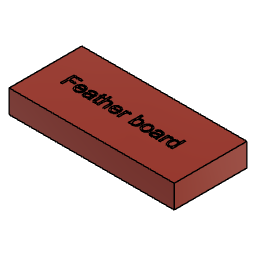
Feather board v1 (Autodesk Fusion 360 design; units mm, degrees)
Autodesk Fusion 360 part; units mm, degrees
sketch "Sketch1" plane through (0, 0, 0) normal (0, 0, 1) x (1, 0, 0)
  line L0 (0, 0) -> (50, 0)
  line L1 (50, 0) -> (50, 22)
  line L2 (50, 22) -> (0, 22)
  line L3 (0, 22) -> (0, 0)
  dimension "d1" = 50
  dimension "d2" = 22
  constraint horizontal L0
  constraint vertical L1
  constraint horizontal L2
  constraint vertical L3
  constraint coincident L0.start L3.end
  measures "d1" distance of L0.start L0.end
  measures "d2" distance of L0.start L2.end
extrude "Extrude1" add sketch "Sketch1" along normal blind 7
sketch "Sketch3" plane through (0, 0, 7) normal (0, 0, 1) x (-1, 0, 0)
  line L0 (0, -22) -> (0, 0)
  line L1 (0, 0) -> (-50, 0)
  line L2 (-50, 0) -> (-50, -22)
  line L3 (-50, -22) -> (0, -22)
  line L4 (-6.3934, -9.8568) -> (-49.9798, -9.3295) construction
  line L5 (-49.9798, -9.3295) -> (-50.0202, -12.6705) construction
  line L6 (-50.0202, -12.6705) -> (-6.4338, -13.1978) construction
  line L7 (-6.4338, -13.1978) -> (-6.3934, -9.8568) construction
  dimension "d5" = 4
  text T0 "Feather board" font "Arial" height 4 align left top in box 43.5896 x 3.3413 at (-6.3934, -9.8568) x (-0.999927, 0.012098) y (-0.012098, -0.999927) spacing 1
  constraint midpoint L2
extrude "Extrude2" cut sketch "Sketch3" against normal blind 1 text T0
